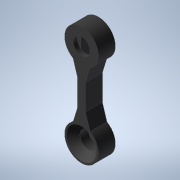
# Autodesk Inventor part: 2nd arm
Saved by Autodesk Inventor 2022 (Build 260153000, 153)
## iProperties
Created: 2022-02-04
Part Number: 2nd arm
Material: Generic
Document SubType Name: Modeling
Designer: Alexa
Density: 1 g/cm^3
Appearance: Default
Author: Alexa
Autodesk Inventor part; units mm, degrees
ref_plane "YZ Plane" through (0, 0, 0) normal (1, 0, 0) x (0, 1, 0)
ref_plane "XZ Plane" through (0, 0, 0) normal (0, 1, 0) x (-1, 0, 0)
ref_plane "XY Plane" through (0, 0, 0) normal (0, 0, 1) x (1, 0, 0)
sketch "Sketch1" plane through (0, 0, 0) normal (0, 0, 1) x (1, 0, 0)
  circle A0 centre (0, 0) radius 10
  circle A1 centre (0, 0) radius 30
  line L0 (0, 0) -> (10, 0)
  line L1 (10, 0) -> (10, 100)
  line L2 (10, 100) -> (0, 100)
  line L3 (0, 100) -> (0, 0)
  line L4 (0, 100) -> (-10, 100)
  line L5 (-10, 100) -> (-10, 0)
  line L6 (-10, 0) -> (0, 0)
  line L7 (0, 0) -> (0, 100)
  circle A2 centre (0, 100) radius 30
  circle A3 centre (0, 100) radius 10
  circle A4 centre (0, 0) radius 20
  circle A5 centre (0, 100) radius 20
  point P0 (10, 17.3205)
  point P1 (10, 82.6795)
  point P2 (-10, 82.6795)
  point P3 (-10, 17.3205)
  dimension "d0" = 20
  dimension "d1" = 60
  dimension "d2" = 10
  dimension "d3" = 100
  dimension "d4" = 60
  dimension "d5" = 40
  dimension "d6" = 40
  constraints: 16 end point, 6 coincident, 4 centre point, 4 parallel, 2 horizontal, 2 horizontal alignment, 2 perpendicular, 1 point on line, 4 other
  measures "d1" diameter of A1
  measures "d2" distance of L2.end L1.end
  measures "d3" distance of L1.end L0.end
  measures "d4" diameter of A2
  measures "d5" diameter of A4
  measures "d6" diameter of A5
extrude "Extrusion1" add sketch "Sketch1" along normal blind 20 contours L5 A4 L3 A0 | A0 L1 A4 L5 | A0 L3 A4 L1 | L5 A1 L3 A4 | A4 L3 A1 L1 | L5 A2 L3 A1 | A1 L3 A2 L1 | L5 A5 L3 A2 | A2 L3 A5 L1 | A5 L1 A3 L5 | L5 A3 L3 A5 | A5 L3 A3 L1 | A3 L2 L4 | L4 L3 A3 | A3 L3 L2
sketch "Sketch2" plane through (0, 0, 20) normal (0, 0, 1) x (1, 0, 0)
  circle A0 centre (0, 100) radius 10
  point P0 (0, 0)
  dimension "d9" = 20
  constraints: 1 centre point
  measures "d9" diameter of A0
extrude "Extrusion2" cut sketch "Sketch2" against normal blind 5
sketch "Sketch3" plane through (0, 0, 0) normal (0, 0, -1) x (-1, 0, 0)
  line L0 (0, 100) -> (6, 100)
  line L1 (6, 100) -> (6, 83)
  line L2 (6, 83) -> (0, 83)
  line L3 (0, 83) -> (0, 100)
  line L4 (0, 100) -> (-6, 100)
  line L5 (-6, 100) -> (-6, 83)
  line L6 (-6, 83) -> (0, 83)
  line L7 (0, 83) -> (0, 100)
  line L8 (6, 100) -> (-6, 100)
  line L9 (-6, 100) -> (-6, 106)
  line L10 (-6, 106) -> (6, 106)
  line L11 (6, 106) -> (6, 100)
  point P0 (0, 0)
  dimension "d12" = 6
  dimension "d13" = 17
  dimension "d14" = 6
  dimension "d15" = 6
  constraints: 24 end point, 6 parallel, 3 horizontal, 3 perpendicular, 2 point on line
  measures "d12" distance of L1.end L2.end
  measures "d13" distance of L0.end L1.end
  measures "d14" distance of L6.end L5.end
  measures "d15" distance of L8.end L9.end
extrude "Extrusion3" cut sketch "Sketch3" against normal blind 15
sketch "Sketch4" plane through (0, 0, 0) normal (0, 0, -1) x (-1, 0, 0)
  line L0 (6, 83) -> (-6, 83)
  line L1 (-6, 83) -> (-6, 78.3)
  line L2 (-6, 78.3) -> (6, 78.3)
  line L3 (6, 78.3) -> (6, 83)
  line L4 (6, 106) -> (-6, 106) projected
  line L5 (6, 106) -> (-6, 106)
  line L6 (-6, 106) -> (-6, 110.7)
  line L7 (-6, 110.7) -> (6, 110.7)
  line L8 (6, 110.7) -> (6, 106)
  point P0 (0, 0)
  dimension "d18" = 12
  dimension "d19" = 4.7
  dimension "d20" = 4.7
  constraints: 16 end point, 4 parallel, 2 horizontal, 2 perpendicular, 1 point on line
  measures "d18" distance of L2.end L1.end
  measures "d19" distance of L1.end L0.end
  measures "d20" distance of L5.end L6.end
extrude "Extrusion4" cut sketch "Sketch4" against normal blind 11.5
sketch "Sketch5" plane through (0, 0, 11.5) normal (0, 0, -1) x (-1, 0, 0)
  line L0 (6, 110.7) -> (6, 78.3) projected
  line L1 (-6, 78.3) -> (-6, 110.7) projected
  line L2 (6, 110.7) -> (-6, 110.7)
  line L3 (-6, 110.7) -> (-6, 108.4)
  line L4 (-6, 108.4) -> (6, 108.4)
  line L5 (6, 108.4) -> (6, 110.7)
  line L6 (6, 78.2245) -> (-6, 78.2245)
  line L7 (-6, 78.2245) -> (-6, 80.5245)
  line L8 (-6, 80.5245) -> (6, 80.5245)
  line L9 (6, 80.5245) -> (6, 78.2245)
  circle A0 centre (0, 108.4) radius 0.75
  circle A1 centre (0, 80.5245) radius 0.75
  point P0 (0, 0)
  dimension "d23" = 2.3
  dimension "d24" = 2.3
  dimension "d25" = 1.5
  dimension "d26" = 1.5
  constraints: 16 end point, 4 parallel, 3 point on line, 2 centre point, 2 horizontal, 2 midpoint, 2 perpendicular
  measures "d23" distance of L3.end L2.end
  measures "d24" distance of L6.end L7.end
  measures "d25" diameter of A0
  measures "d26" diameter of A1
extrude "Extrusion5" cut sketch "Sketch5" against normal blind 48.975 contours A0 L4 | L4 A0 | A1 L8 | L8 A1
sketch "Sketch6" plane through (0, 0, 0) normal (0, 0, -1) x (-1, 0, 0)
  circle A0 centre (0, 0) radius 10
  constraints: 1 centre point, 1 coincident
extrude "Extrusion6" add sketch "Sketch6" against normal blind 2
sketch "Sketch7" plane through (0, 0, 0) normal (0, 0, -1) x (-1, 0, 0)
  circle A0 centre (0, 0) radius 1.5
  circle A1 centre (0, 7) radius 1.5
  circle A2 centre (0, -7) radius 1.5
  dimension "d31" = 3
  dimension "d32" = 3
  dimension "d33" = 3
  constraints: 3 centre point, 1 coincident
  measures "d31" diameter of A0
  measures "d32" diameter of A1
  measures "d33" diameter of A2
extrude "Extrusion7" cut sketch "Sketch7" against normal blind 10.7
chamfer "Chamfer1" distance 8 angle 45 1 edges at (-10, 0, 20)
sketch "Sketch8" plane through (0, 0, 20) normal (0, 0, 1) x (1, 0, 0)
  line L0 (-10, 82.6795) -> (-10, 17.3205) projected
  line L1 (10, 17.3205) -> (10, 82.6795) projected
  line L2 (-10, 82.6795) -> (10, 17.3205)
  line L3 (10, 17.3205) -> (10, 82.6795)
  arc A0 (-10, 17.3205) -> (10, 17.3205) centre (0, 0) ccw projected
  line L4 (10, 82.6795) -> (-10, 17.3205)
  line L5 (-10, 17.3205) -> (-10, 82.6795)
  line L6 (0, 50) -> (4.6328, 50)
  line L7 (4.6328, 50) -> (4.6328, 65.1396)
  line L8 (4.6328, 65.1396) -> (0, 65.1396)
  line L9 (0, 65.1396) -> (0, 50)
  line L10 (0, 50) -> (4.6328, 50)
  line L11 (4.6328, 50) -> (4.6328, 34.8604)
  line L12 (4.6328, 34.8604) -> (0, 34.8604)
  line L13 (0, 34.8604) -> (0, 50)
  line L14 (4.6328, 34.8604) -> (-4.6328, 34.8604)
  line L15 (-4.6328, 34.8604) -> (-4.6328, 65.1396)
  line L16 (-4.6328, 65.1396) -> (4.6328, 65.1396)
  line L17 (4.6328, 65.1396) -> (4.6328, 34.8604)
  constraints: 32 end point, 8 equal length, 3 horizontal, 3 perpendicular, 3 point on line, 1 midpoint
extrude "Extrusion8" cut sketch "Sketch8" against normal blind 38.5125 contours L2 L15 L4 L0 | L2 L11 L7 L4 L1
body "Solid1"
